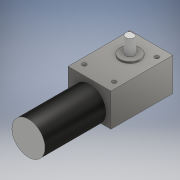
# Autodesk Inventor part: motor
Saved by Autodesk Inventor 2017 (Build 210142000, 142)
## iProperties
Created: 2018-01-02
Part Number: motor
Material: Generic
Document SubType Name: Modeling
Designer: RLanting
Density: 1 g/cm^3
Appearance: Default
Author: RLanting
Autodesk Inventor part; units mm, degrees
ref_plane "YZ Plane" through (0, 0, 0) normal (1, 0, 0) x (0, 1, 0)
ref_plane "XZ Plane" through (0, 0, 0) normal (0, 1, 0) x (-1, 0, 0)
sketch "Sketch1" plane through (0, 0, 0) normal (0, 0, 1) x (1, 0, 0)
  line L0 (20.06, -29.05) -> (-20.06, -29.05)
  line L1 (-20.06, -29.05) -> (-20.06, 29.05)
  line L2 (-20.06, 29.05) -> (20.06, 29.05)
  line L3 (20.06, 29.05) -> (20.06, -29.05)
  line L4 (20.06, -29.05) -> (-20.06, 29.05) construction
  line L5 (-20.06, -29.05) -> (20.06, 29.05) construction
  point P0 (0, 0)
  dimension "d0" = 40.12
  dimension "d1" = 58.1
  constraints: 12 end point, 2 midpoint, 2 parallel, 1 horizontal, 1 perpendicular
  measures "d0" distance of L1.end L2.end
  measures "d1" distance of L2.end L0.start
extrude "Extrusion1" add sketch "Sketch1" along normal blind 31
sketch "Sketch2" plane through (0, 0, 31) normal (0, 0, 1) x (1, 0, 0)
  line L0 (0, 0) -> (0, 8.85) construction
  circle A0 centre (0, 8.85) radius 9.4
  line L1 (-20.06, -29.05) -> (20.06, -29.05) projected
  dimension "d4" = 18.8
  dimension "d5" = 37.9
  constraints: 2 end point, 1 centre point, 1 coincident, 1 vertical
  measures "d4" diameter of A0
  measures "d5" distance from line of L0.end L1
extrude "Extrusion2" add sketch "Sketch2" along normal blind 1.5
sketch "Sketch3" plane through (0, 8.85, 32.5) normal (0, 0, 1) x (1, 0, 0)
  circle A0 centre (0, 0) radius 9.4 projected
  circle A1 centre (0, 0) radius 4
  point P0 (0, -8.85)
  dimension "d8" = 8
  constraints: 1 centre point, 1 coincident
  measures "d8" diameter of A1
extrude "Extrusion3" add sketch "Sketch3" along normal blind 14.9 contours A1
sketch "Sketch4" plane through (0, 8.85, 47.4) normal (0, 0, 1) x (1, 0, 0)
  circle A0 centre (0, 0) radius 4 construction
  arc A1 (2.6458, 3) -> (-2.6458, 3) centre (0, 0) ccw
  line L0 (-2.6458, 3) -> (2.6458, 3)
  point P0 (0, -8.85)
  dimension "d11" = 7
  constraints: 2 end point, 2 point on circle, 1 centre point, 1 coincident, 1 horizontal, 2 other
extrude "Extrusion4" cut sketch "Sketch4" against normal blind 12
sketch "Sketch5" plane through (0, 0, 31) normal (0, 0, 1) x (1, 0, 0)
  circle A0 centre (0, 8.85) radius 9.4 construction
  line L0 (-20.06, -29.05) -> (20.06, -29.05) construction
  line L1 (20.06, -29.05) -> (20.06, 29.05) construction
  line L2 (20.06, 29.05) -> (-20.06, 29.05) construction
  line L3 (-20.06, 29.05) -> (-20.06, -29.05) construction
  line L4 (0, 29.05) -> (0, -29.05) construction
  line L5 (-20.06, -29.05) -> (20.06, -29.05) construction
  line L6 (14, -20) -> (-14, -20) construction
  line L7 (-14, -20) -> (-14, 20) construction
  line L8 (-14, 20) -> (14, 20) construction
  line L9 (14, 20) -> (14, -20) construction
  line L10 (14, -20) -> (-14, 20) construction
  line L11 (-14, -20) -> (14, 20) construction
  circle A1 centre (-14, 20) radius 2
  circle A2 centre (14, 20) radius 2
  circle A3 centre (14, -20) radius 2
  circle A4 centre (-14, -20) radius 2
  point P0 (0, 0)
  dimension "d14" = 28
  dimension "d15" = 40
  dimension "d16" = 4
  constraints: 14 end point, 4 centre point, 4 coincident, 4 midpoint, 3 equal radius, 2 parallel, 1 horizontal, 1 perpendicular
  measures "d14" distance of L7.end L8.end
  measures "d15" distance of L6.end L7.end
  measures "d16" diameter of A1
extrude "Extrusion5" cut sketch "Sketch5" against normal blind 6
ref_plane "Work Plane1" through (0, 0, 15.5) normal (0, 0, 1) x (1, 0, 0)
mirror "Mirror1" about plane through (0, 0, 15.5) normal (0, 0, 1) of "Extrusion5", "Extrusion2"
sketch "Sketch6" plane through (-20.06, -29.05, 0) normal (0, -1, 0) x (1, 0, 0)
  line L0 (20.06, 0) -> (20.06, 11.3) construction
  circle A0 centre (20.06, 11.3) radius 15.5
  line L1 (40.12, 0) -> (0, 0) projected
  point P0 (20.06, -4.2)
  dimension "d19" = 31
  dimension "d20" = 4.2
  constraints: 2 end point, 2 vertical alignment, 1 coincident, 1 midpoint, 1 vertical, 2 other
  measures "d20" distance from line of point (20.06, -4.2) L1
extrude "Extrusion6" add sketch "Sketch6" along normal blind 57.2
body "Solid1"
